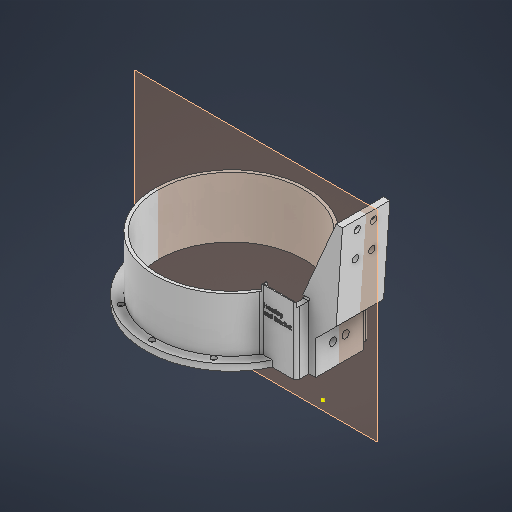
# Autodesk Inventor part: Holder_and_Cylinder
Saved by Autodesk Inventor 2026 (Build 300175000, 175)
## iProperties
Created: 2025-06-26
Part Number: Holder_and_Cylinder
Material: Generic
Document SubType Name: Modeling
Designer: Charl
Density: 1 g/cm^3
Appearance: Default
Author: Charl
Autodesk Inventor part; units mm, degrees
(part 1 of 2)
ref_plane "YZ Plane" through (0, 0, 0) normal (1, 0, 0) x (0, 1, 0)
ref_plane "XZ Plane" through (0, 0, 0) normal (0, 1, 0) x (-1, 0, 0)
ref_plane "XY Plane" through (0, 0, 0) normal (0, 0, 1) x (1, 0, 0)
sketch "Sketch1" plane through (0, 0, 0) normal (0, 1, 0) x (-1, 0, 0)
  circle A0 centre (0, 0) radius 135
  circle A1 centre (0, 0) radius 120
  dimension "d0" = 270
  dimension "d1" = 240
  constraints: 2 centre point, 2 coincident
  measures "d0" diameter of A0
  measures "d1" diameter of A1
extrude "Extrusion1" add sketch "Sketch1" along normal blind 10
sketch "Sketch2" plane through (0, 10, 0) normal (0, 1, 0) x (1, 0, 0)
  circle A0 centre (0, 0) radius 115.125
  circle A1 centre (0, 0) radius 120
  dimension "d4" = 230.25
  constraints: 2 centre point, 2 coincident
  measures "d4" diameter of A0
extrude "Extrusion2" add sketch "Sketch2" along normal blind 85.5 and the other way blind 10
sketch "Sketch3" plane through (0, 10, 0) normal (0, 1, 0) x (1, 0, 0)
  line L0 (70.125, 57.5) -> (160.125, 57.5)
  line L1 (160.125, 57.5) -> (160.125, -57.5)
  line L2 (160.125, -57.5) -> (70.125, -57.5)
  line L3 (70.125, -57.5) -> (70.125, 57.5)
  line L4 (71.625, 56) -> (158.625, 56)
  line L5 (158.625, 56) -> (158.625, -56)
  line L6 (158.625, -56) -> (71.625, -56)
  line L7 (71.625, -56) -> (71.625, 56)
  line L8 (-160.125, 32.5) -> (-70.125, 32.5)
  line L9 (-70.125, 32.5) -> (-70.125, -32.5)
  line L10 (-70.125, -32.5) -> (-160.125, -32.5)
  line L11 (-160.125, -32.5) -> (-160.125, 32.5)
  line L12 (-158.625, 31) -> (-71.625, 31)
  line L13 (-71.625, 31) -> (-71.625, -31)
  line L14 (-71.625, -31) -> (-158.625, -31)
  line L15 (-158.625, -31) -> (-158.625, 31)
  line L16 (-150.359, 85.157) -> (-65.125, 85.157)
  line L17 (-65.125, 85.157) -> (-65.125, 46.3)
  line L18 (-65.125, 46.3) -> (-150.359, 46.3)
  line L19 (-150.359, 46.3) -> (-150.359, 85.157)
  line L20 (-148.359, 83.157) -> (-67.125, 83.157)
  line L21 (-67.125, 83.157) -> (-67.125, 48.3)
  line L22 (-67.125, 48.3) -> (-148.359, 48.3)
  line L23 (-148.359, 48.3) -> (-148.359, 83.157)
  line L24 (-150.359, -46.3) -> (-65.125, -46.3)
  line L25 (-65.125, -46.3) -> (-65.125, -85.157)
  line L26 (-65.125, -85.157) -> (-150.359, -85.157)
  line L27 (-150.359, -85.157) -> (-150.359, -46.3)
  line L28 (-148.359, -48.3) -> (-67.125, -48.3)
  line L29 (-67.125, -48.3) -> (-67.125, -83.157)
  line L30 (-67.125, -83.157) -> (-148.359, -83.157)
  line L31 (-148.359, -83.157) -> (-148.359, -48.3)
  circle A0 centre (0, 0) radius 134.272
  circle A1 centre (0, 0) radius 132.2722
  circle A2 centre (0, 0) radius 115.125
  circle A3 centre (0, 0) radius 120
  point P0 (70.125, 0)
  point P1 (121.3372, 57.5)
  point P2 (122.0368, 56)
  point P3 (122.0368, -56)
  point P4 (121.3372, -57.5)
  point P5 (106.132, 56)
  point P6 (100.5871, 56)
  point P7 (100.5871, -56)
  point P8 (106.132, -56)
  point P9 (105.3269, 57.5)
  point P10 (105.3269, -57.5)
  dimension "d7" = 90
  dimension "d8" = 115
  dimension "d9" = 57.5
  dimension "d10" = 70.125
  dimension "d11" = 1.5
  dimension "d12" = 1.5
  dimension "d13" = 1.5
  dimension "d14" = 1.5
  dimension "d15" = 90
  dimension "d16" = 65
  dimension "d17" = 32.5
  dimension "d18" = 70.125
  dimension "d19" = 1.5
  dimension "d20" = 1.5
  dimension "d21" = 1.5
  dimension "d22" = 1.5
  dimension "d23" = 85.234
  dimension "d24" = 38.857
  dimension "d25" = 2
  dimension "d26" = 2
  dimension "d27" = 2
  dimension "d28" = 2
  dimension "d29" = 65.125
  dimension "d30" = 13.8
  dimension "d31" = 13.8
  dimension "d32" = 65.125
  dimension "d33" = 38.857
  dimension "d34" = 85.234
  dimension "d35" = 2
  dimension "d36" = 2
  dimension "d37" = 2
  dimension "d38" = 2
  dimension "d39" = 268.544
  dimension "d40" = 264.5444
  dimension "d42" = 230.25
  dimension "d45" = 240
  constraints: 64 end point, 16 parallel, 8 horizontal, 8 perpendicular, 4 centre point, 3 coincident, 1 midpoint
  measures "d7" distance of L0.start L0.end
  measures "d8" distance of L0.end L1.end
  measures "d9" distance from line of point (0, 0) L0
  measures "d10" distance of point (70.125, 0) point (0, 0)
  measures "d11" distance between parallel lines of L1 L5
  measures "d12" distance between parallel lines of L2 L6
  measures "d13" distance between parallel lines of L0 L4
  measures "d14" distance between parallel lines of L3 L7
  measures "d15" distance of L8.start L8.end
  measures "d16" distance of L8.end L9.end
  measures "d17" distance from line of point (0, 0) L8
  measures "d18" distance from line of L9 point (0, 0)
  measures "d19" distance between parallel lines of L10 L14
  measures "d20" distance between parallel lines of L9 L13
  measures "d21" distance between parallel lines of L8 L12
  measures "d22" distance between parallel lines of L11 L15
  measures "d23" distance of L17.end L18.end
  measures "d24" distance of L16.end L17.end
  measures "d25" distance between parallel lines of L16 L20
  measures "d26" distance between parallel lines of L19 L23
  measures "d27" distance between parallel lines of L18 L22
  measures "d28" distance between parallel lines of L17 L21
  measures "d29" distance from line of point (0, 0) L17
  measures "d30" distance from line of L8 L18.end
  measures "d31" distance between parallel lines of L10 L24
  measures "d32" distance from line of point (0, 0) L25
  measures "d33" distance of L26.end L24.start
  measures "d34" distance of L25.end L26.end
  measures "d35" distance between parallel lines of L27 L31
  measures "d36" distance between parallel lines of L24 L28
  measures "d37" distance between parallel lines of L25 L29
  measures "d38" distance between parallel lines of L26 L30
  measures "d39" diameter of A0
  measures "d40" diameter of A1
  measures "d42" diameter of A2
  measures "d45" diameter of A3
extrude "Extrusion3" cut sketch "Sketch3" along normal mid plane 85.5 contours L0 L1 L2 A0 L6 L5 L4
extrude "Extrusion4" cut sketch "Sketch3" along normal blind 85.5 contours L4 A3 L6 A2
extrude "Extrusion5" add sketch "Sketch3" along normal blind 85.5 and the other way blind 10 contours L0 A1 L4 A3 | L0 A0 L4 A1 | A3 L6 A1 L2 | L0 L1 L2 A0 L6 L5 L4 | A1 L6 A0 L2
sketch "Sketch5" plane through (0, 0, 0) normal (0, -1, 0) x (1, 0, 0)
  line L0 (135, -56) -> (160, -56)
  line L1 (160, -56) -> (160, 56)
  line L2 (160, 56) -> (135, 56)
  line L3 (135, 56) -> (135, -56)
  arc A0 (122.8373, -56) -> (122.8373, 56) centre (0, 0) ccw projected
  dimension "d57" = 25
  dimension "d58" = 112
  dimension "d59" = 56
  constraints: 8 end point, 2 parallel, 1 horizontal, 1 perpendicular, 1 tangent
  measures "d57" distance of L0.start L0.end
  measures "d58" distance of L2.end L0.start
  measures "d59" distance from line of point (0, 0) L0
extrude "Extrusion7" add sketch "Sketch5" against normal blind 80
chamfer "Chamfer1" distance 40 angle 23.25 1 edges at (135, 80, 0) measured on face at (135, 79.5, 0)
ref_plane "Work Plane1" through (105.3269, 10, 0) normal (0, 0, 1) x (1, 0, 0)
sketch "Sketch6" plane through (135, 40, -56) normal (-0.9187912, 0.3947439, 0) x (0, 0, 1)
  circle A0 centre (56, 33.7805) radius 5.5
  circle A1 centre (56, 33.7805) radius 2
  circle A2 centre (46, 10.0805) radius 5.5
  circle A3 centre (46, 10.0805) radius 2
  line L0 (56, 109.6115) -> (56, -231.2929) projected
  line L1 (112, 43.5355) -> (0, 43.5355) projected
  circle A4 centre (66, 10.0805) radius 5.5
  circle A5 centre (66, 10.0805) radius 2
  point P0 (56, -90.0421)
  dimension "d65" = 11
  dimension "d66" = 4
  dimension "d67" = 11
  dimension "d68" = 4
  dimension "d69" = 10
  dimension "d70" = 23.7
  dimension "d71" = 9.755
  dimension "d72" = 11
  dimension "d73" = 4
  dimension "d76" = 23.7
  dimension "d77" = 10
  constraints: 6 centre point, 3 coincident
  measures "d65" diameter of A0
  measures "d66" diameter of A1
  measures "d67" diameter of A2
  measures "d68" diameter of A3
  measures "d69" distance from line of L0 A2.centre
  measures "d70" vertical distance of A0.centre A2.centre
  measures "d71" distance from line of L1 A0.centre
  measures "d72" diameter of A4
  measures "d73" diameter of A5
  measures "d76" vertical distance of A0.centre A4.centre
  measures "d77" distance from line of A5.centre L0
extrude "Extrusion8" cut sketch "Sketch6" against normal blind 55 contours A0 L0 A1 | L0 A1 A0 | L0 A1 | A1 L0 | A2 | A3 | A4 | A5
extrude "Extrusion9" add sketch "Sketch6" against normal blind 5 contours A0 L0 A1 | L0 A1 A0 | A2 | A4
sketch "Sketch17" plane through (160.125, 0, -57.5) normal (1, 0, 0) x (0, 0, -1)
  line L0 (-95, 111) -> (-20, 111)
  line L1 (-20, 111) -> (-20, 76)
  line L2 (-20, 76) -> (-95, 76)
  line L3 (-95, 76) -> (-95, 111)
  line L4 (-115, 0) -> (-115, 95.5) projected
  line L5 (-115, 95.5) -> (0, 95.5) projected
  point P0 (-57.5, 0)
  dimension "d130" = 20
  dimension "d131" = 35
  dimension "d132" = 19.5
  dimension "d133" = 75
  constraints: 8 end point, 2 parallel, 1 horizontal, 1 perpendicular
  measures "d130" distance between parallel lines of L4 L3
  measures "d131" distance between parallel lines of L2 L0
  measures "d132" distance between parallel lines of L5 L2
  measures "d133" distance between parallel lines of L1 L3
extrude "Extrusion16" cut sketch "Sketch17" against normal blind 40.5
sketch "Sketch18" plane through (0, 95.5, 0) normal (0, 1, 0) x (1, 0, 0)
  line L0 (100.5871, 56) -> (158.625, 56) projected
  line L1 (152.1854, 37.5) -> (152.1854, 56) projected
  line L2 (158.625, 56) -> (152.1854, 56)
  line L3 (152.1854, 56) -> (152.1854, 37.5)
  line L4 (152.1854, 37.5) -> (158.625, 37.5)
  line L5 (158.625, 37.5) -> (158.625, 56)
  line L6 (160.125, -37.5) -> (150.4668, -37.5) projected
  line L7 (158.625, -56) -> (100.5871, -56) projected
  line L8 (152.1854, -37.5) -> (158.625, -37.5)
  line L9 (158.625, -37.5) -> (158.625, -56)
  line L10 (158.625, -56) -> (152.1854, -56)
  line L11 (152.1854, -56) -> (152.1854, -37.5)
  point P0 (0, 0)
  constraints: 16 end point, 4 parallel, 2 horizontal, 2 perpendicular, 2 point on line
extrude "Extrusion17" add sketch "Sketch18" against normal blind 40.5
sketch "Sketch19" plane through (0, 95.5, 0) normal (0, 1, 0) x (1, 0, 0)
  arc A0 (105.3269, 57.5) -> (105.3269, -57.5) centre (0, 0) ccw projected
  line L0 (152.1854, 56) -> (135, 56) projected
  line L1 (106.132, 56) -> (152.1854, 56)
  line L2 (106.132, 56) -> (106.132, 57.5)
  line L3 (105.3269, 57.5) -> (122.1423, 57.5) projected
  line L4 (160.125, 57.5) -> (160.125, -57.5) projected
  line L5 (106.132, 57.5) -> (160.125, 57.5)
  line L6 (160.125, 57.5) -> (160.125, -57.5)
  line L7 (160.125, -57.5) -> (106.132, -57.5)
  line L8 (106.132, -57.5) -> (106.132, -56)
  line L9 (135, -56) -> (152.1854, -56) projected
  line L10 (152.1854, -56) -> (106.132, -56)
  line L11 (152.1854, -37.5) -> (150.4668, -37.5) projected
  line L12 (152.1854, -56) -> (152.1854, -37.5)
  line L13 (152.1854, -37.5) -> (160.125, -37.5)
  line L14 (122.726, 57.5) -> (142.726, 57.5)
  line L15 (142.726, 57.5) -> (142.726, 56)
  line L16 (142.726, 56) -> (122.726, 56)
  line L17 (122.726, 56) -> (122.726, 57.5)
  line L18 (152.1854, 56) -> (152.1854, 37.5) projected
  line L19 (152.1854, 56) -> (152.1854, 37.5)
  line L20 (152.1854, 37.5) -> (160.125, 37.5)
  dimension "d138" = 20
  dimension "d139" = 17.399
  constraints: 30 end point, 6 point on line, 5 perpendicular, 3 horizontal, 3 vertical, 2 collinear, 2 parallel
  measures "d138" distance of L15.end L16.end
  measures "d139" distance between parallel lines of L4 L15
extrude "Extrusion18" add sketch "Sketch19" along normal blind 4 contours L0 L15 L5 L4 L20 L18 | L1 L2 L3 L5 L17 | L4 L7 L8 L10 L9 L12 L13
sketch "Sketch20" plane through (122.8373, 10, 56) normal (0, 0, -1) x (-1, 0, 0)
  line L0 (-29.3481, 89.5) -> (-29.3481, 70) projected
  line L1 (16.7053, 85.5) -> (16.7053, 89.5) projected
  line L2 (-29.3481, 89.5) -> (16.7053, 89.5)
  line L3 (16.7053, 89.5) -> (16.7053, 88)
  line L4 (16.7053, 88) -> (-29.3481, 88)
  line L5 (-29.3481, 88) -> (-29.3481, 89.5)
  point P0 (122.8373, -10)
  dimension "d142" = 1.5
  constraints: 8 end point, 2 parallel, 1 horizontal, 1 perpendicular, 1 point on line
  measures "d142" distance of L2.end L3.end
extrude "Extrusion19" add sketch "Sketch20" along normal blind 5
sketch "Sketch21" plane through (0, 99.5, 0) normal (0, 1, 0) x (1, 0, 0)
  line L0 (106.132, 57.5) -> (106.132, 56) projected
  line L1 (106.132, 57.5) -> (107.632, 57.5)
  line L2 (107.632, 57.5) -> (107.632, 51)
  line L3 (107.632, 51) -> (106.132, 51)
  line L4 (106.132, 51) -> (106.132, 57.5)
  line L5 (160.125, -57.5) -> (122.1423, -57.5) projected
  line L6 (106.132, -56) -> (106.132, -51) projected
  line L7 (160.125, -57.5) -> (106.132, -57.5)
  line L8 (106.132, -57.5) -> (106.132, -56)
  line L9 (106.132, -56) -> (160.125, -56)
  line L10 (160.125, -56) -> (160.125, -57.5)
  point P0 (0, 0)
  dimension "d145" = 1.5
  dimension "d146" = 6.5
  dimension "d147" = 1.5
  constraints: 16 end point, 4 parallel, 2 horizontal, 2 perpendicular
  measures "d145" distance of L2.end L3.end
  measures "d146" distance of L1.end L2.end
  measures "d147" distance of L7.end L6.start
extrude "Extrusion20" add sketch "Sketch21" along normal blind 6.5
sketch "Sketch22" plane through (160.125, 99.5, 56) normal (0, 0, -1) x (-1, 0, 0)
  line L0 (412.3732, -43.6088) -> (412.3732, -42.1088)
  line L1 (412.3732, -42.1088) -> (412.3732, -42.1088)
  line L2 (0, -99.5) -> (0, 6.5) projected
  line L3 (53.993, -4) -> (53.993, 6.5) projected
  line L4 (0, 6.5) -> (53.993, 6.5)
  line L5 (53.993, 6.5) -> (53.993, 5)
  line L6 (53.993, 5) -> (0, 5)
  line L7 (0, 5) -> (0, 6.5)
  line L8 (53.993, 0) -> (0, 0) projected
  line L9 (53.993, 6.5) -> (52.493, 6.5)
  line L10 (52.493, 6.5) -> (52.493, 0)
  line L11 (52.493, 0) -> (53.993, 0)
  line L12 (53.993, 0) -> (53.993, 6.5)
  point P0 (160.125, -99.5)
  dimension "d150" = 1.5
  dimension "d151" = 1.5
  dimension "d152" = 1.5
  constraints: 20 end point, 4 parallel, 3 horizontal, 2 perpendicular, 2 point on line, 2 vertical, 5 other
  measures "d150" distance of L0.end L0.start
  measures "d151" distance of L4.end L5.end
  measures "d152" distance of L11.end L10.end
extrude "Extrusion21" add sketch "Sketch22" along normal blind 5 contours L10 L6 L3 L8 | L10 L4 L3 L6
sketch "Sketch23" plane through (106.132, 10, -56) normal (0, 0, 1) x (1, 0, 0)
  line L0 (16.594, 85.5) -> (16.594, 89.5) projected
  line L1 (0, 85.5) -> (0, 89.5) projected
  line L2 (16.594, 89.5) -> (0, 89.5)
  line L3 (0, 89.5) -> (0, 88)
  line L4 (0, 88) -> (16.594, 88)
  line L5 (16.594, 88) -> (16.594, 89.5)
  line L6 (36.594, 89.5) -> (46.0534, 89.5) projected
  line L7 (46.0534, 70) -> (46.0534, 89.5) projected
  line L8 (36.594, 89.5) -> (46.0534, 89.5)
  line L9 (46.0534, 89.5) -> (46.0534, 88)
  line L10 (46.0534, 88) -> (36.594, 88)
  line L11 (36.594, 88) -> (36.594, 89.5)
  point P0 (-106.132, -10)
  dimension "d155" = 1.5
  dimension "d156" = 1.5
  constraints: 16 end point, 4 parallel, 2 horizontal, 2 perpendicular, 2 point on line
  measures "d155" distance of L3.end L2.end
  measures "d156" distance of L8.end L9.end
extrude "Extrusion22" add sketch "Sketch23" along normal blind 5
sketch "Sketch24" plane through (107.632, 99.5, -51) normal (1, 0, 0) x (0, 0, -1)
  line L0 (0, 0) -> (0, 6.5) projected
  line L1 (6.5, 0) -> (6.5, 6.5) projected
  line L2 (0, 6.5) -> (6.5, 6.5)
  line L3 (6.5, 6.5) -> (6.5, 5)
  line L4 (6.5, 5) -> (0, 5)
  line L5 (0, 5) -> (0, 6.5)
  point P0 (-51, -99.5)
  point P1 (0, 5)
  dimension "d159" = 1.5
  constraints: 8 end point, 2 parallel, 1 horizontal, 1 perpendicular, 1 point on line
  measures "d159" distance of L2.end L3.end
extrude "Extrusion23" add sketch "Sketch24" along normal blind 5
fillet "Fillet2" radius 5 6 edges at (100.5871, 52.75, 56) (100.5871, 52.75, -56) (105.3269, 52.75, -57.5) (105.3269, 52.75, 57.5) (160.125, 49.75, -57.5) (160.125, 53, 57.5)
chamfer "Chamfer2" distance 4 angle 45 2 edges at (129.1587, 98, 56) (152.1854, 98, 53.5)
ref_plane "Work Plane2" through (135, 0, 56) normal (-0.4107189, -0.911762, 0) x (0, 0, -1)
sketch "Sketch27" plane through (0, 0, 0) normal (0, -1, 0) x (1, 0, 0)
  line L0 (152.1854, 51) -> (152.1854, 56) projected
  line L1 (122.726, -56) -> (106.132, -56) projected
  line L2 (152.1854, 56) -> (121.3527, 56)
  line L3 (121.3527, 56) -> (121.3527, -56)
  line L4 (121.3527, -56) -> (152.1854, -56)
  line L5 (152.1854, -56) -> (152.1854, 56)
  point P0 (0, 0)
  constraints: 8 end point, 2 parallel, 1 horizontal, 1 perpendicular, 1 point on line
extrude "Extrusion25" add sketch "Sketch27" against normal blind 10
sketch "Sketch25" plane through (135, 0, 56) normal (-0.4107189, -0.911762, 0) x (0, 0, -1)
  line L0 (18.5, -17.1126) -> (93.5, -17.1126) projected
  circle A0 centre (56, -31.1821) radius 20
  ellipse E0 centre (56, -127.1951) end of major axis (-59.125, -127.1951) minor radius 104.9666 (114.461, -36.7692) -> (-2.461, -36.7692) ccw projected
  point P0 (56, -123.0879)
  dimension "d170" = 40
  dimension "d172" = 96.013
  constraints: 1 centre point, 1 other
  measures "d170" diameter of A0
  measures "d172" distance of point (56, -127.195) A0.centre
extrude "Extrusion24" cut sketch "Sketch25" along normal mid plane 80
sketch "Sketch28" plane through (0, 10, 0) normal (0, 1, 0) x (1, 0, 0)
  circle A0 centre (0, 0) radius 125
  circle A1 centre (0, 0) radius 135
  circle A2 centre (0, 125) radius 2.75
  circle A3 centre (0, 125) radius 4.35
  dimension "d177" = 250
  dimension "d178" = 270
  dimension "d179" = 5.5
  dimension "d180" = 8.7
  constraints: 3 centre point, 3 coincident, 1 vertical alignment, 2 other
  measures "d178" diameter of A1
  measures "d179" diameter of A2
  measures "d180" diameter of A3
extrude "Extrusion26" cut sketch "Sketch28" against normal blind 5 contours A3 A0 A2 | A0 A2 A3 | A2 A0 | A0 A2
extrude "Extrusion27" cut sketch "Sketch28" against normal blind 10 contours A2 A0 | A0 A2
pattern_circular "Circular Pattern1" count 10 over 360 about axis through (0, 0, 0) along (0, 1, 0) of "Extrusion26", "Extrusion27"
sketch "Sketch29" plane through (160.125, 76, 37.5) normal (0, 1, 0) x (1, 0, 0)
  line L0 (-9.6582, 75) -> (-7.9396, 75) projected
  line L1 (-9.6582, 75) -> (10.6418, 75)
  line L2 (10.6418, 75) -> (10.6418, 0)
  line L3 (10.6418, 0) -> (-9.6582, 0)
  line L4 (-9.6582, 0) -> (-9.6582, 75)
  point P0 (-160.125, 37.5)
  point P1 (-7.9396, 75)
  dimension "d188" = 75
  dimension "d189" = 20.3
  constraints: 8 end point, 2 parallel, 1 horizontal, 1 perpendicular
  measures "d188" distance of L1.end L2.end
  measures "d189" distance of L2.end L3.end
extrude "HolderStart" add sketch "Sketch29" along normal blind 10 separate body
sketch "Sketch31" plane through (160.125, 76, 37.5) normal (0, -1, 0) x (1, 0, 0)
  line L0 (-9.6582, 0) -> (10.6418, 0) projected
  line L1 (0, -75) -> (0, 0) projected
  line L2 (10.6418, 0) -> (0, 0)
  line L3 (0, 0) -> (0, -75)
  line L4 (0, -75) -> (10.6418, -75)
  line L5 (10.6418, -75) -> (10.6418, 0)
  point P0 (-160.125, -37.5)
  constraints: 8 end point, 2 parallel, 1 horizontal, 1 perpendicular
extrude "Extrusion30" add sketch "Sketch31" along normal blind 76 bodies 2
sketch "Sketch32" plane through (150.4668, 86, 37.5) normal (0, 0, 1) x (1, 0, 0)
  line L0 (20.3, -86) -> (20.3, 0) projected
  line L1 (52.705, 0) -> (115.8158, 0) construction
  line L2 (0, 0) -> (20.3, 0) projected
  line L3 (0, 0) -> (0, 13.494)
  line L4 (8.2289, 20) -> (-42.8348, 20) projected
  line L5 (0, 13.494) -> (10, 13.494)
  line L6 (10, 13.494) -> (10, 17.494)
  line L7 (10, 17.494) -> (0, 17.494)
  line L8 (20.3, -32.405) -> (52.705, 0)
  line L9 (0, 17.494) -> (14.8386, 52.0317)
  line L10 (14.8386, 52.0317) -> (16.9363, 56.9144)
  line L11 (52.705, 0) -> (52.705, 74.2114) construction
  line L12 (52.705, 74.2114) -> (52.705, 193.2478) construction
  line L13 (16.9363, 56.9144) -> (52.705, 140.1682)
  line L14 (52.705, 116.8926) -> (42.705, 116.8926)
  line L15 (42.705, 116.8926) -> (42.705, 116.8926) construction
  line L16 (52.705, 116.8926) -> (62.705, 116.8926) construction
  line L17 (62.705, 116.8926) -> (134.3375, 116.8926) construction
  line L18 (52.705, 140.1682) -> (62.705, 140.1682)
  line L19 (62.705, 140.1682) -> (52.705, 0)
  point P0 (-150.4668, -86)
  dimension "d200" = 13.494
  dimension "d201" = 4
  dimension "d211" = 45
  dimension "d212" = 0
  dimension "d213" = 32.405
  dimension "d239" = 10
  dimension "d240" = 10
  dimension "d241" = 66.75
  dimension "d244" = 10
  dimension "d245" = 0
  dimension "d246" = 66.75
  dimension "d247" = 10
  constraints: 34 end point, 6 perpendicular, 5 point on line, 3 horizontal, 2 vertical
  measures "d200" distance of L2.start L3.end
  measures "d201" distance of L5.end L6.end
  measures "d211" angle of L8 L0
  measures "d212" vertical distance of L0.end L1.start
  measures "d213" distance of L0.end L8.start
  measures "d239" distance of L6.end L7.end
  measures "d240" distance of L3.end L5.end
  measures "d241" angle of L7 L9
  measures "d244" distance of L14.start L14.end
  measures "d245" distance of L14.end L15.end
  measures "d246" angle of L1 L13
  measures "d247" distance of L14.start L16.end
extrude "Extrusion35" add sketch "Sketch32" against normal blind 75 bodies 2
ref_plane "Work Plane7" through (150.4668, 103.494, 37.5) normal (0.3947439, 0.9187912, 0) x (0, 0, -1)
sketch "Sketch35" plane through (150.4668, 103.494, 37.5) normal (0.3947439, 0.9187912, 0) x (0, 0, -1)
  line L0 (0, 0) -> (75, 0) projected
  circle A0 centre (37.5, 15) radius 35
  point P0 (37.5, 97.394)
  dimension "d252" = 70
  dimension "d253" = 15
  constraints: 1 centre point
  measures "d252" diameter of A0
  measures "d253" distance from line of L0 A0.centre
extrude "Extrusion36" cut sketch "Sketch35" along normal blind 67.371 and the other way blind 65.75 bodies 2
ref_plane "Work Plane9" through (166.2261, 2.0933, -37.5) normal (-0.9081432, 0.4186597, 0) x (0, 0, 1)
ref_plane "Work Plane8" through (170.7668, 0, -37.5) normal (-0.9081432, 0.4186597, 0) x (0, 0, 1)
sketch "Sketch36" plane through (166.2261, 2.0933, -37.5) normal (-0.9081432, 0.4186597, 0) x (0, 0, 1)
  circle A0 centre (50.5, 208.9598) radius 2
  circle A1 centre (50.5, 208.9598) radius 5
  circle A2 centre (50.5, 169.9598) radius 2
  circle A3 centre (50.5, 169.9598) radius 5
  line L0 (75, 91.667) -> (0, 91.667) construction
  line L1 (37.5, -67.9361) -> (37.5, 251.2701) construction
  circle A4 centre (24.5, 208.9598) radius 2
  circle A5 centre (24.5, 208.9598) radius 5
  circle A6 centre (24.5, 169.9598) radius 2
  circle A7 centre (24.5, 169.9598) radius 5
  line L2 (75, 223.1464) -> (0, 223.1464) projected
  line L3 (75, 218.9598) -> (0, 218.9598) projected
  point P0 (37.5, -71.4932)
  point P1 (37.5, 91.667)
  dimension "d260" = 10
  dimension "d261" = 4
  dimension "d262" = 10
  dimension "d263" = 4
  dimension "d264" = 39
  dimension "d266" = 26
  dimension "d267" = 10
  dimension "d268" = 26
  constraints: 8 centre point, 4 coincident, 4 symmetric about line, 2 end point, 2 midpoint, 1 vertical, 4 other
  measures "d260" diameter of A1
  measures "d261" diameter of A0
  measures "d262" diameter of A3
  measures "d263" diameter of A2
  measures "d264" distance of A2.centre A0.centre
  measures "d266" distance of A5.centre A0.centre
  measures "d267" distance from line of L3 A0.centre
  measures "d268" distance of A7.centre A2.centre
extrude "Extrusion37" cut sketch "Sketch36" along normal blind 49 contours A0 | A1 | A2 | A3 | A4 | A5 | A6 | A7 bodies 2
extrude "Extrusion38" cut sketch "Sketch36" along normal blind 75 contours A0 | A2 | A4 | A6 bodies 2
ref_plane "Work Plane10" through (196.4064, 56.2628, -37.5) normal (-0.9187912, 0.3947439, 0) x (0, 0, 1)
sketch "Sketch37" plane through (196.4064, 56.2628, -37.5) normal (-0.9187912, 0.3947439, 0) x (0, 0, 1)
  point P0 (37.5, -129.224)
sketch "Sketch38" plane through (196.4064, 56.2628, -37.5) normal (-0.9187912, 0.3947439, 0) x (0, 0, 1)
  circle A0 centre (47.5, -29.1015) radius 5.5 projected
  circle A1 centre (27.5, -29.1015) radius 5.5 projected
  circle A2 centre (37.5, -5.4015) radius 5.5 projected
  circle A3 centre (27.5, -29.1015) radius 5.5
  circle A4 centre (47.5, -29.1015) radius 5.5
  circle A5 centre (37.5, -5.4015) radius 5.5
  point P0 (37.5, -129.224)
  constraints: 3 centre point, 3 coincident, 3 concentric
extrude "Extrusion39" cut sketch "Sketch38" along normal blind 44.5 bodies 2
sketch "Sketch39" plane through (122.1423, 0, 57.5) normal (0, 0, 1) x (1, 0, 0)
  line L0 (-13.5441, 81.6413) -> (29.5653, 81.6413) construction
  line L1 (29.5653, 81.6413) -> (29.5653, 47.1733) construction
  line L2 (29.5653, 47.1733) -> (-13.5441, 47.1733) construction
  line L3 (-13.5441, 47.1733) -> (-13.5441, 81.6413) construction
  line L4 (-8.497, 75.5017) -> (-9.3077, 75.5017)
  line L5 (-9.3077, 75.5017) -> (-9.3077, 78.4875)
  line L6 (-9.3077, 78.4875) -> (-12.1155, 78.4875)
  line L7 (-12.1155, 78.4875) -> (-12.1155, 75.5017)
  line L8 (-12.1155, 75.5017) -> (-12.9262, 75.5017)
  line L9 (-12.9262, 75.5017) -> (-12.9262, 81.6017)
  line L10 (-12.9262, 81.6017) -> (-12.1155, 81.6017)
  line L11 (-12.1155, 81.6017) -> (-12.1155, 79.2092)
  line L12 (-12.1155, 79.2092) -> (-9.3077, 79.2092)
  line L13 (-9.3077, 79.2092) -> (-9.3077, 81.6017)
  line L14 (-9.3077, 81.6017) -> (-8.497, 81.6017)
  line L15 (-8.497, 81.6017) -> (-8.497, 75.5017)
  spline S0 degree 2 poles (-3.5587, 77.7905) (-3.5587, 76.6337) (-4.6709, 75.3732) (-5.6002, 75.3732) knots 0 0 0 1 2 2 2
  spline S1 degree 2 poles (-5.6002, 75.3732) (-6.5543, 75.3732) (-7.6468, 76.6733) (-7.6468, 77.7905) knots 0 0 0 1 2 2 2
  spline S2 degree 2 poles (-7.6468, 77.7905) (-7.6468, 78.9373) (-6.5197, 80.2077) (-5.6002, 80.2077) knots 0 0 0 1 2 2 2
  spline S3 degree 2 poles (-5.6002, 80.2077) (-4.6709, 80.2077) (-3.5587, 78.9423) (-3.5587, 77.7905) knots 0 0 0 1 2 2 2
  spline S4 degree 2 poles (-4.3545, 77.7905) (-4.3545, 78.6803) (-5.0021, 79.5453) (-5.6002, 79.5453) knots 0 0 0 1 2 2 2
  spline S5 degree 2 poles (-5.6002, 79.5453) (-6.1984, 79.5453) (-6.8509, 78.6803) (-6.8509, 77.7905) knots 0 0 0 1 2 2 2
  spline S6 degree 2 poles (-6.8509, 77.7905) (-6.8509, 76.9254) (-6.1984, 76.0356) (-5.6002, 76.0356) knots 0 0 0 1 2 2 2
  spline S7 degree 2 poles (-5.6002, 76.0356) (-5.007, 76.0356) (-4.3545, 76.9106) (-4.3545, 77.7905) knots 0 0 0 1 2 2 2
  line L16 (0.7914, 75.5017) -> (0.0203, 75.5017)
  line L17 (0.0203, 75.5017) -> (0.0203, 76.0059)
  spline S8 degree 2 poles (0.0203, 76.0059) (-0.3357, 75.6945) (-0.9733, 75.3732) (-1.3688, 75.3732) knots 0 0 0 1 2 2 2
  spline S9 degree 2 poles (-1.3688, 75.3732) (-1.6654, 75.3732) (-2.1943, 75.5709) (-2.3871, 75.7835) knots 0 0 0 1 2 2 2
  spline S10 degree 2 poles (-2.3871, 75.7835) (-2.5848, 75.9961) (-2.8023, 76.6436) (-2.8023, 77.1083) knots 0 0 0 1 2 2 2
  line L18 (-2.8023, 77.1083) -> (-2.8023, 80.0792)
  line L19 (-2.8023, 80.0792) -> (-2.0312, 80.0792)
  line L20 (-2.0312, 80.0792) -> (-2.0312, 77.4692)
  spline S11 degree 2 poles (-2.0312, 77.4692) (-2.0312, 77.1034) (-1.9768, 76.6239) (-1.8829, 76.4459) knots 0 0 0 1 2 2 2
  spline S12 degree 2 poles (-1.8829, 76.4459) (-1.789, 76.2679) (-1.4677, 76.1048) (-1.1661, 76.1048) knots 0 0 0 1 2 2 2
  spline S13 degree 2 poles (-1.1661, 76.1048) (-0.8844, 76.1048) (-0.2467, 76.4261) (0.0203, 76.6585) knots 0 0 0 1 2 2 2
  line L21 (0.0203, 76.6585) -> (0.0203, 80.0792)
  line L22 (0.0203, 80.0792) -> (0.7914, 80.0792)
  line L23 (0.7914, 80.0792) -> (0.7914, 75.5017)
  spline S14 degree 2 poles (3.1444, 75.393) (2.6847, 75.393) (1.8888, 75.6401) (1.6268, 75.7786) knots 0 0 0 1 2 2 2
  line L24 (1.6268, 75.7786) -> (1.6268, 76.6436)
  line L25 (1.6268, 76.6436) -> (1.6664, 76.6436)
  spline S15 degree 2 poles (1.6664, 76.6436) (1.7652, 76.5645) (2.0322, 76.3767) (2.2546, 76.2729) knots 0 0 0 1 2 2 2
  spline S16 degree 2 poles (2.2546, 76.2729) (2.4474, 76.179) (2.922, 76.0405) (3.1741, 76.0405) knots 0 0 0 1 2 2 2
  spline S17 degree 2 poles (3.1741, 76.0405) (3.357, 76.0405) (3.7771, 76.1246) (3.876, 76.1938) knots 0 0 0 1 2 2 2
  spline S18 degree 2 poles (3.876, 76.1938) (4.0194, 76.2877) (4.1479, 76.5003) (4.1479, 76.7178) knots 0 0 0 1 2 2 2
  spline S19 degree 2 poles (4.1479, 76.7178) (4.1479, 76.9897) (3.8513, 77.2714) (3.4707, 77.3653) knots 0 0 0 1 2 2 2
  spline S20 degree 2 poles (3.4707, 77.3653) (3.3224, 77.3999) (2.8478, 77.4988) (2.6451, 77.5532) knots 0 0 0 1 2 2 2
  spline S21 degree 2 poles (2.6451, 77.5532) (2.1212, 77.7064) (1.6466, 78.3392) (1.6466, 78.789) knots 0 0 0 1 2 2 2
  spline S22 degree 2 poles (1.6466, 78.789) (1.6466, 79.4119) (2.5809, 80.188) (3.352, 80.188) knots 0 0 0 1 2 2 2
  spline S23 degree 2 poles (3.352, 80.188) (3.7327, 80.188) (4.5038, 80.0001) (4.7658, 79.8568) knots 0 0 0 1 2 2 2
  line L26 (4.7658, 79.8568) -> (4.7658, 79.0312)
  line L27 (4.7658, 79.0312) -> (4.7263, 79.0312)
  spline S24 degree 2 poles (4.7263, 79.0312) (4.4297, 79.2685) (3.7079, 79.5404) (3.3372, 79.5404) knots 0 0 0 1 2 2 2
  spline S25 degree 2 poles (3.3372, 79.5404) (2.9566, 79.5404) (2.4326, 79.2191) (2.4326, 78.8978) knots 0 0 0 1 2 2 2
  spline S26 degree 2 poles (2.4326, 78.8978) (2.4326, 78.6061) (2.744, 78.3243) (3.09, 78.2354) knots 0 0 0 1 2 2 2
  spline S27 degree 2 poles (3.09, 78.2354) (3.2581, 78.1909) (3.6832, 78.1019) (3.9156, 78.0475) knots 0 0 0 1 2 2 2
  spline S28 degree 2 poles (3.9156, 78.0475) (4.4198, 77.919) (4.9339, 77.3307) (4.9339, 76.8216) knots 0 0 0 1 2 2 2
  spline S29 degree 2 poles (4.9339, 76.8216) (4.9339, 76.525) (4.7015, 76.001) (4.4742, 75.8082) knots 0 0 0 1 2 2 2
  spline S30 degree 2 poles (4.4742, 75.8082) (4.2319, 75.6055) (3.614, 75.393) (3.1444, 75.393) knots 0 0 0 1 2 2 2
  line L28 (6.4366, 75.5017) -> (5.6655, 75.5017)
  line L29 (5.6655, 75.5017) -> (5.6655, 80.0792)
  line L30 (5.6655, 80.0792) -> (6.4366, 80.0792)
  line L31 (6.4366, 80.0792) -> (6.4366, 75.5017)
  line L32 (6.491, 80.8405) -> (5.616, 80.8405)
  line L33 (5.616, 80.8405) -> (5.616, 81.6413)
  line L34 (5.616, 81.6413) -> (6.491, 81.6413)
  line L35 (6.491, 81.6413) -> (6.491, 80.8405)
  line L36 (11.1624, 75.5017) -> (10.3912, 75.5017)
  line L37 (10.3912, 75.5017) -> (10.3912, 78.1118)
  spline S31 degree 2 poles (10.3912, 78.1118) (10.3912, 78.4282) (10.3319, 78.9719) (10.243, 79.135) knots 0 0 0 1 2 2 2
  spline S32 degree 2 poles (10.243, 79.135) (10.149, 79.3081) (9.8129, 79.4761) (9.5262, 79.4761) knots 0 0 0 1 2 2 2
  spline S33 degree 2 poles (9.5262, 79.4761) (9.2395, 79.4761) (8.6314, 79.1696) (8.3398, 78.9225) knots 0 0 0 1 2 2 2
  line L38 (8.3398, 78.9225) -> (8.3398, 75.5017)
  line L39 (8.3398, 75.5017) -> (7.5686, 75.5017)
  line L40 (7.5686, 75.5017) -> (7.5686, 80.0792)
  line L41 (7.5686, 80.0792) -> (8.3398, 80.0792)
  line L42 (8.3398, 80.0792) -> (8.3398, 79.57)
  spline S34 degree 2 poles (8.3398, 79.57) (8.6858, 79.8815) (9.3532, 80.2077) (9.7289, 80.2077) knots 0 0 0 1 2 2 2
  spline S35 degree 2 poles (9.7289, 80.2077) (10.4011, 80.2077) (11.1624, 79.3179) (11.1624, 78.4726) knots 0 0 0 1 2 2 2
  line L43 (11.1624, 78.4726) -> (11.1624, 75.5017)
  spline S36 degree 2 poles (12.4081, 74.7701) (12.4872, 74.7355) (12.7887, 74.6268) (12.9815, 74.5823) knots 0 0 0 1 2 2 2
  spline S37 degree 2 poles (12.9815, 74.5823) (13.1941, 74.5279) (13.5549, 74.4636) (13.7675, 74.4636) knots 0 0 0 1 2 2 2
  spline S38 degree 2 poles (13.7675, 74.4636) (14.1234, 74.4636) (14.6177, 74.6515) (14.7562, 74.8196) knots 0 0 0 1 2 2 2
  spline S39 degree 2 poles (14.7562, 74.8196) (14.8896, 74.9876) (14.9934, 75.4276) (14.9934, 75.7093) knots 0 0 0 1 2 2 2
  line L44 (14.9934, 75.7093) -> (14.9934, 76.1098)
  spline S40 degree 2 poles (14.9934, 76.1098) (14.682, 75.8379) (14.0839, 75.5808) (13.634, 75.5808) knots 0 0 0 1 2 2 2
  spline S41 degree 2 poles (13.634, 75.5808) (12.853, 75.5808) (11.9286, 76.7425) (11.9286, 77.835) knots 0 0 0 1 2 2 2
  spline S42 degree 2 poles (11.9286, 77.835) (11.9286, 78.4034) (12.2499, 79.2833) (12.5169, 79.5948) knots 0 0 0 1 2 2 2
  spline S43 degree 2 poles (12.5169, 79.5948) (12.7739, 79.8864) (13.4808, 80.2077) (13.8565, 80.2077) knots 0 0 0 1 2 2 2
  spline S44 degree 2 poles (13.8565, 80.2077) (14.2124, 80.2077) (14.7314, 80.0397) (14.9934, 79.8864) knots 0 0 0 1 2 2 2
  line L45 (14.9934, 79.8864) -> (15.0379, 80.0792)
  line L46 (15.0379, 80.0792) -> (15.7646, 80.0792)
  line L47 (15.7646, 80.0792) -> (15.7646, 76.0257)
  spline S45 degree 2 poles (15.7646, 76.0257) (15.7646, 74.8591) (14.7512, 73.7716) (13.7082, 73.7716) knots 0 0 0 1 2 2 2
  spline S46 degree 2 poles (13.7082, 73.7716) (13.372, 73.7716) (12.6701, 73.8803) (12.3686, 73.9693) knots 0 0 0 1 2 2 2
  line L48 (12.3686, 73.9693) -> (12.3686, 74.7701)
  line L49 (12.3686, 74.7701) -> (12.4081, 74.7701)
  line L50 (14.9934, 76.7425) -> (14.9934, 79.2586)
  spline S47 degree 2 poles (14.9934, 79.2586) (14.7067, 79.397) (14.2223, 79.5157) (13.9801, 79.5157) knots 0 0 0 1 2 2 2
  spline S48 degree 2 poles (13.9801, 79.5157) (13.3968, 79.5157) (12.7245, 78.6555) (12.7245, 77.8498) knots 0 0 0 1 2 2 2
  spline S49 degree 2 poles (12.7245, 77.8498) (12.7245, 77.0885) (13.2336, 76.2927) (13.8071, 76.2927) knots 0 0 0 1 2 2 2
  spline S50 degree 2 poles (13.8071, 76.2927) (14.1086, 76.2927) (14.7413, 76.5299) (14.9934, 76.7425) knots 0 0 0 1 2 2 2
  spline S51 degree 2 poles (-10.4348, 65.9427) (-10.5287, 65.8735) (-10.8451, 65.6263) (-10.9934, 65.5522) knots 0 0 0 1 2 2 2
  spline S52 degree 2 poles (-10.9934, 65.5522) (-11.196, 65.4434) (-11.5767, 65.3297) (-11.9227, 65.3297) knots 0 0 0 1 2 2 2
  spline S53 degree 2 poles (-11.9227, 65.3297) (-12.2045, 65.3297) (-12.7136, 65.5423) (-12.9064, 65.7351) knots 0 0 0 1 2 2 2
  spline S54 degree 2 poles (-12.9064, 65.7351) (-13.0893, 65.9229) (-13.3117, 66.4766) (-13.3117, 66.783) knots 0 0 0 1 2 2 2
  spline S55 degree 2 poles (-13.3117, 66.783) (-13.3117, 67.2576) (-12.9113, 67.9299) (-12.4763, 68.1227) knots 0 0 0 1 2 2 2
  spline S56 degree 2 poles (-12.4763, 68.1227) (-12.0908, 68.3006) (-11.0428, 68.4341) (-10.4348, 68.4687) knots 0 0 0 1 2 2 2
  line L51 (-10.4348, 68.4687) -> (-10.4348, 68.617)
  spline S57 degree 2 poles (-10.4348, 68.617) (-10.4348, 68.8839) (-10.5979, 69.2151) (-10.7462, 69.3091) knots 0 0 0 1 2 2 2
  spline S58 degree 2 poles (-10.7462, 69.3091) (-10.8945, 69.403) (-11.3196, 69.4623) (-11.547, 69.4623) knots 0 0 0 1 2 2 2
  spline S59 degree 2 poles (-11.547, 69.4623) (-11.8139, 69.4623) (-12.5357, 69.3041) (-12.8965, 69.1509) knots 0 0 0 1 2 2 2
  line L52 (-12.8965, 69.1509) -> (-12.941, 69.1509)
  line L53 (-12.941, 69.1509) -> (-12.941, 69.9368)
  spline S60 degree 2 poles (-12.941, 69.9368) (-12.7284, 69.9962) (-11.9326, 70.1445) (-11.5421, 70.1445) knots 0 0 0 1 2 2 2
  spline S61 degree 2 poles (-11.5421, 70.1445) (-11.0675, 70.1445) (-10.4199, 69.9962) (-10.1629, 69.8034) knots 0 0 0 1 2 2 2
  spline S62 degree 2 poles (-10.1629, 69.8034) (-9.9108, 69.6155) (-9.6636, 69.0174) (-9.6636, 68.5873) knots 0 0 0 1 2 2 2
  line L54 (-9.6636, 68.5873) -> (-9.6636, 65.4582)
  line L55 (-9.6636, 65.4582) -> (-10.4348, 65.4582)
  line L56 (-10.4348, 65.4582) -> (-10.4348, 65.9427)
  line L57 (-10.4348, 66.5853) -> (-10.4348, 67.8557)
  spline S63 degree 2 poles (-10.4348, 67.8557) (-10.7116, 67.831) (-11.547, 67.747) (-11.809, 67.6679) knots 0 0 0 1 2 2 2
  spline S64 degree 2 poles (-11.809, 67.6679) (-12.1155, 67.574) (-12.5159, 67.1834) (-12.5159, 66.8374) knots 0 0 0 1 2 2 2
  spline S65 degree 2 poles (-12.5159, 66.8374) (-12.5159, 66.442) (-12.071, 66.0415) (-11.6459, 66.0415) knots 0 0 0 1 2 2 2
  spline S66 degree 2 poles (-11.6459, 66.0415) (-11.285, 66.0415) (-10.6918, 66.353) (-10.4348, 66.5853) knots 0 0 0 1 2 2 2
  line L58 (-4.9873, 65.4582) -> (-5.7584, 65.4582)
  line L59 (-5.7584, 65.4582) -> (-5.7584, 68.0683)
  spline S67 degree 2 poles (-5.7584, 68.0683) (-5.7584, 68.3847) (-5.8177, 68.9284) (-5.9067, 69.0915) knots 0 0 0 1 2 2 2
  spline S68 degree 2 poles (-5.9067, 69.0915) (-6.0006, 69.2646) (-6.3368, 69.4326) (-6.6235, 69.4326) knots 0 0 0 1 2 2 2
  spline S69 degree 2 poles (-6.6235, 69.4326) (-6.9102, 69.4326) (-7.5182, 69.1262) (-7.8099, 68.879) knots 0 0 0 1 2 2 2
  line L60 (-7.8099, 68.879) -> (-7.8099, 65.4582)
  line L61 (-7.8099, 65.4582) -> (-8.581, 65.4582)
  line L62 (-8.581, 65.4582) -> (-8.581, 70.0357)
  line L63 (-8.581, 70.0357) -> (-7.8099, 70.0357)
  line L64 (-7.8099, 70.0357) -> (-7.8099, 69.5266)
  spline S70 degree 2 poles (-7.8099, 69.5266) (-7.4639, 69.838) (-6.7965, 70.1642) (-6.4208, 70.1642) knots 0 0 0 1 2 2 2
  spline S71 degree 2 poles (-6.4208, 70.1642) (-5.7485, 70.1642) (-4.9873, 69.2744) (-4.9873, 68.4291) knots 0 0 0 1 2 2 2
  line L65 (-4.9873, 68.4291) -> (-4.9873, 65.4582)
  line L66 (-0.3851, 65.4582) -> (-1.1562, 65.4582)
  line L67 (-1.1562, 65.4582) -> (-1.1562, 65.9229)
  spline S72 degree 2 poles (-1.1562, 65.9229) (-1.3342, 65.7746) (-1.5962, 65.5769) (-1.7741, 65.4928) knots 0 0 0 1 2 2 2
  spline S73 degree 2 poles (-1.7741, 65.4928) (-1.9373, 65.4138) (-2.2882, 65.3297) (-2.5206, 65.3297) knots 0 0 0 1 2 2 2
  spline S74 degree 2 poles (-2.5206, 65.3297) (-2.8963, 65.3297) (-3.529, 65.6411) (-3.7515, 65.9427) knots 0 0 0 1 2 2 2
  spline S75 degree 2 poles (-3.7515, 65.9427) (-3.9739, 66.2442) (-4.2211, 67.134) (-4.2211, 67.7124) knots 0 0 0 1 2 2 2
  spline S76 degree 2 poles (-4.2211, 67.7124) (-4.2211, 68.3155) (-3.9096, 69.1954) (-3.6378, 69.5266) knots 0 0 0 1 2 2 2
  spline S77 degree 2 poles (-3.6378, 69.5266) (-3.3857, 69.8232) (-2.6788, 70.1642) (-2.2882, 70.1642) knots 0 0 0 1 2 2 2
  spline S78 degree 2 poles (-2.2882, 70.1642) (-1.9472, 70.1642) (-1.438, 70.011) (-1.1562, 69.8528) knots 0 0 0 1 2 2 2
  line L68 (-1.1562, 69.8528) -> (-1.1562, 71.8301)
  line L69 (-1.1562, 71.8301) -> (-0.3851, 71.8301)
  line L70 (-0.3851, 71.8301) -> (-0.3851, 65.4582)
  line L71 (-1.1562, 66.5705) -> (-1.1562, 69.2151)
  spline S79 degree 2 poles (-1.1562, 69.2151) (-1.4429, 69.3535) (-1.8977, 69.4574) (-2.1597, 69.4574) knots 0 0 0 1 2 2 2
  spline S80 degree 2 poles (-2.1597, 69.4574) (-2.7529, 69.4574) (-3.4252, 68.5676) (-3.4252, 67.7272) knots 0 0 0 1 2 2 2
  spline S81 degree 2 poles (-3.4252, 67.7272) (-3.4252, 66.9165) (-2.9111, 66.0613) (-2.3426, 66.0613) knots 0 0 0 1 2 2 2
  spline S82 degree 2 poles (-2.3426, 66.0613) (-2.0411, 66.0613) (-1.4281, 66.3381) (-1.1562, 66.5705) knots 0 0 0 1 2 2 2
  spline S83 degree 2 poles (7.5489, 67.3317) (7.5489, 66.877) (7.2028, 66.18) (6.9161, 65.9526) knots 0 0 0 1 2 2 2
  spline S84 degree 2 poles (6.9161, 65.9526) (6.5701, 65.6856) (5.7841, 65.4582) (5.1613, 65.4582) knots 0 0 0 1 2 2 2
  line L72 (5.1613, 65.4582) -> (3.4113, 65.4582)
  line L73 (3.4113, 65.4582) -> (3.4113, 71.5582)
  line L74 (3.4113, 71.5582) -> (5.0278, 71.5582)
  spline S85 degree 2 poles (5.0278, 71.5582) (5.6803, 71.5582) (6.3328, 71.4742) (6.6294, 71.3111) knots 0 0 0 1 2 2 2
  spline S86 degree 2 poles (6.6294, 71.3111) (6.9606, 71.1381) (7.2622, 70.5696) (7.2622, 70.184) knots 0 0 0 1 2 2 2
  spline S87 degree 2 poles (7.2622, 70.184) (7.2622, 69.7539) (6.8074, 69.0718) (6.407, 68.879) knots 0 0 0 1 2 2 2
  line L75 (6.407, 68.879) -> (6.407, 68.8493)
  spline S88 degree 2 poles (6.407, 68.8493) (6.9507, 68.701) (7.5489, 67.915) (7.5489, 67.3317) knots 0 0 0 1 2 2 2
  spline S89 degree 2 poles (6.7036, 67.2971) (6.7036, 67.6432) (6.5058, 68.0881) (6.2092, 68.2462) knots 0 0 0 1 2 2 2
  spline S90 degree 2 poles (6.2092, 68.2462) (6.0165, 68.3451) (5.5617, 68.4044) (5.1415, 68.4044) knots 0 0 0 1 2 2 2
  line L76 (5.1415, 68.4044) -> (4.222, 68.4044)
  line L77 (4.222, 68.4044) -> (4.222, 66.1503)
  line L78 (4.222, 66.1503) -> (4.8795, 66.1503)
  spline S91 degree 2 poles (4.8795, 66.1503) (5.4134, 66.1503) (6.0263, 66.2492) (6.2636, 66.4074) knots 0 0 0 1 2 2 2
  spline S92 degree 2 poles (6.2636, 66.4074) (6.491, 66.5705) (6.7036, 66.9758) (6.7036, 67.2971) knots 0 0 0 1 2 2 2
  spline S93 degree 2 poles (6.4169, 70.0703) (6.4169, 70.2878) (6.2686, 70.6141) (6.1054, 70.708) knots 0 0 0 1 2 2 2
  spline S94 degree 2 poles (6.1054, 70.708) (5.9077, 70.8168) (5.4282, 70.8662) (4.9981, 70.8662) knots 0 0 0 1 2 2 2
  line L79 (4.9981, 70.8662) -> (4.222, 70.8662)
  line L80 (4.222, 70.8662) -> (4.222, 69.0817)
  line L81 (4.222, 69.0817) -> (5.1415, 69.0817)
  spline S95 degree 2 poles (5.1415, 69.0817) (5.5221, 69.0817) (5.883, 69.1608) (6.0758, 69.2843) knots 0 0 0 1 2 2 2
  spline S96 degree 2 poles (6.0758, 69.2843) (6.2636, 69.403) (6.4169, 69.7836) (6.4169, 70.0703) knots 0 0 0 1 2 2 2
  line L82 (10.7224, 69.2102) -> (10.6829, 69.2102)
  spline S97 degree 2 poles (10.6829, 69.2102) (10.5939, 69.2349) (10.4011, 69.2448) (10.2677, 69.2448) knots 0 0 0 1 2 2 2
  spline S98 degree 2 poles (10.2677, 69.2448) (9.9562, 69.2448) (9.3433, 68.9729) (9.0665, 68.706) knots 0 0 0 1 2 2 2
  line L83 (9.0665, 68.706) -> (9.0665, 65.4582)
  line L84 (9.0665, 65.4582) -> (8.2953, 65.4582)
  line L85 (8.2953, 65.4582) -> (8.2953, 70.0357)
  line L86 (8.2953, 70.0357) -> (9.0665, 70.0357)
  line L87 (9.0665, 70.0357) -> (9.0665, 69.3535)
  spline S99 degree 2 poles (9.0665, 69.3535) (9.4866, 69.7292) (10.1144, 70.0357) (10.411, 70.0357) knots 0 0 0 1 2 2 2
  spline S100 degree 2 poles (10.411, 70.0357) (10.5297, 70.0357) (10.6483, 70.0258) (10.7224, 70.011) knots 0 0 0 1 2 2 2
  line L88 (10.7224, 70.011) -> (10.7224, 69.2102)
  spline S101 degree 2 poles (13.8713, 65.9427) (13.7774, 65.8735) (13.461, 65.6263) (13.3127, 65.5522) knots 0 0 0 1 2 2 2
  spline S102 degree 2 poles (13.3127, 65.5522) (13.1101, 65.4434) (12.7294, 65.3297) (12.3834, 65.3297) knots 0 0 0 1 2 2 2
  spline S103 degree 2 poles (12.3834, 65.3297) (12.1016, 65.3297) (11.5925, 65.5423) (11.3997, 65.7351) knots 0 0 0 1 2 2 2
  spline S104 degree 2 poles (11.3997, 65.7351) (11.2168, 65.9229) (10.9943, 66.4766) (10.9943, 66.783) knots 0 0 0 1 2 2 2
  spline S105 degree 2 poles (10.9943, 66.783) (10.9943, 67.2576) (11.3947, 67.9299) (11.8297, 68.1227) knots 0 0 0 1 2 2 2
  spline S106 degree 2 poles (11.8297, 68.1227) (12.2153, 68.3006) (13.2633, 68.4341) (13.8713, 68.4687) knots 0 0 0 1 2 2 2
  line L89 (13.8713, 68.4687) -> (13.8713, 68.617)
  spline S107 degree 2 poles (13.8713, 68.617) (13.8713, 68.8839) (13.7082, 69.2151) (13.5599, 69.3091) knots 0 0 0 1 2 2 2
  spline S108 degree 2 poles (13.5599, 69.3091) (13.4116, 69.403) (12.9865, 69.4623) (12.7591, 69.4623) knots 0 0 0 1 2 2 2
  spline S109 degree 2 poles (12.7591, 69.4623) (12.4921, 69.4623) (11.7704, 69.3041) (11.4096, 69.1509) knots 0 0 0 1 2 2 2
  line L90 (11.4096, 69.1509) -> (11.3651, 69.1509)
  line L91 (11.3651, 69.1509) -> (11.3651, 69.9368)
  spline S110 degree 2 poles (11.3651, 69.9368) (11.5776, 69.9962) (12.3735, 70.1445) (12.764, 70.1445) knots 0 0 0 1 2 2 2
  spline S111 degree 2 poles (12.764, 70.1445) (13.2386, 70.1445) (13.8861, 69.9962) (14.1432, 69.8034) knots 0 0 0 1 2 2 2
  spline S112 degree 2 poles (14.1432, 69.8034) (14.3953, 69.6155) (14.6425, 69.0174) (14.6425, 68.5873) knots 0 0 0 1 2 2 2
  line L92 (14.6425, 68.5873) -> (14.6425, 65.4582)
  line L93 (14.6425, 65.4582) -> (13.8713, 65.4582)
  line L94 (13.8713, 65.4582) -> (13.8713, 65.9427)
  line L95 (13.8713, 66.5853) -> (13.8713, 67.8557)
  spline S113 degree 2 poles (13.8713, 67.8557) (13.5945, 67.831) (12.7591, 67.747) (12.4971, 67.6679) knots 0 0 0 1 2 2 2
  spline S114 degree 2 poles (12.4971, 67.6679) (12.1906, 67.574) (11.7902, 67.1834) (11.7902, 66.8374) knots 0 0 0 1 2 2 2
  spline S115 degree 2 poles (11.7902, 66.8374) (11.7902, 66.442) (12.2351, 66.0415) (12.6602, 66.0415) knots 0 0 0 1 2 2 2
  spline S116 degree 2 poles (12.6602, 66.0415) (13.0211, 66.0415) (13.6143, 66.353) (13.8713, 66.5853) knots 0 0 0 1 2 2 2
  spline S117 degree 2 poles (17.5442, 65.3544) (17.0696, 65.3544) (16.2836, 65.6461) (16.0019, 65.9427) knots 0 0 0 1 2 2 2
  spline S118 degree 2 poles (16.0019, 65.9427) (15.7201, 66.2343) (15.4087, 67.134) (15.4087, 67.7371) knots 0 0 0 1 2 2 2
  spline S119 degree 2 poles (15.4087, 67.7371) (15.4087, 68.3402) (15.73, 69.2201) (16.0019, 69.5167) knots 0 0 0 1 2 2 2
  spline S120 degree 2 poles (16.0019, 69.5167) (16.2737, 69.8182) (17.0795, 70.1395) (17.5442, 70.1395) knots 0 0 0 1 2 2 2
  spline S121 degree 2 poles (17.5442, 70.1395) (17.9199, 70.1395) (18.6218, 69.927) (18.8937, 69.7885) knots 0 0 0 1 2 2 2
  line L96 (18.8937, 69.7885) -> (18.8937, 68.9235)
  line L97 (18.8937, 68.9235) -> (18.8492, 68.9235)
  spline S122 degree 2 poles (18.8492, 68.9235) (18.7652, 68.9927) (18.5081, 69.1706) (18.3252, 69.2646) knots 0 0 0 1 2 2 2
  spline S123 degree 2 poles (18.3252, 69.2646) (18.1621, 69.3437) (17.7271, 69.4672) (17.5293, 69.4672) knots 0 0 0 1 2 2 2
  spline S124 degree 2 poles (17.5293, 69.4672) (16.9312, 69.4672) (16.2045, 68.5626) (16.2045, 67.7371) knots 0 0 0 1 2 2 2
  spline S125 degree 2 poles (16.2045, 67.7371) (16.2045, 66.9313) (16.9065, 66.0267) (17.5293, 66.0267) knots 0 0 0 1 2 2 2
  spline S126 degree 2 poles (17.5293, 66.0267) (17.905, 66.0267) (18.5872, 66.3381) (18.8492, 66.5804) knots 0 0 0 1 2 2 2
  line L98 (18.8492, 66.5804) -> (18.8937, 66.5804)
  line L99 (18.8937, 66.5804) -> (18.8937, 65.7153)
  spline S127 degree 2 poles (18.8937, 65.7153) (18.78, 65.6609) (18.434, 65.5077) (18.2955, 65.4731) knots 0 0 0 1 2 2 2
  spline S128 degree 2 poles (18.2955, 65.4731) (18.0978, 65.4138) (17.7864, 65.3544) (17.5442, 65.3544) knots 0 0 0 1 2 2 2
  line L100 (23.3871, 65.4582) -> (22.3737, 65.4582)
  line L101 (22.3737, 65.4582) -> (20.6733, 67.6679)
  line L102 (20.6733, 67.6679) -> (20.3668, 67.3713)
  line L103 (20.3668, 67.3713) -> (20.3668, 65.4582)
  line L104 (20.3668, 65.4582) -> (19.5956, 65.4582)
  line L105 (19.5956, 65.4582) -> (19.5956, 71.8301)
  line L106 (19.5956, 71.8301) -> (20.3668, 71.8301)
  line L107 (20.3668, 71.8301) -> (20.3668, 68.1029)
  line L108 (20.3668, 68.1029) -> (22.176, 70.0357)
  line L109 (22.176, 70.0357) -> (23.135, 70.0357)
  line L110 (23.135, 70.0357) -> (21.2566, 68.1227)
  line L111 (21.2566, 68.1227) -> (23.3871, 65.4582)
  spline S129 degree 2 poles (25.7599, 65.3544) (24.6625, 65.3544) (23.4563, 66.5853) (23.4563, 67.7223) knots 0 0 0 1 2 2 2
  spline S130 degree 2 poles (23.4563, 67.7223) (23.4563, 68.8394) (24.6279, 70.1642) (25.572, 70.1642) knots 0 0 0 1 2 2 2
  spline S131 degree 2 poles (25.572, 70.1642) (25.9972, 70.1642) (26.6546, 69.9171) (26.8968, 69.6551) knots 0 0 0 1 2 2 2
  spline S132 degree 2 poles (26.8968, 69.6551) (27.144, 69.3931) (27.406, 68.6368) (27.406, 68.0881) knots 0 0 0 1 2 2 2
  line L112 (27.406, 68.0881) -> (27.406, 67.6679)
  line L113 (27.406, 67.6679) -> (24.2374, 67.6679)
  spline S133 degree 2 poles (24.2374, 67.6679) (24.2374, 66.872) (25.0382, 66.0267) (25.75, 66.0267) knots 0 0 0 1 2 2 2
  spline S134 degree 2 poles (25.75, 66.0267) (26.0021, 66.0267) (26.4915, 66.1404) (26.6892, 66.2294) knots 0 0 0 1 2 2 2
  spline S135 degree 2 poles (26.6892, 66.2294) (26.8968, 66.3283) (27.1836, 66.5013) (27.2775, 66.5804) knots 0 0 0 1 2 2 2
  line L114 (27.2775, 66.5804) -> (27.322, 66.5804)
  line L115 (27.322, 66.5804) -> (27.322, 65.74)
  spline S136 degree 2 poles (27.322, 65.74) (27.1885, 65.6856) (26.7831, 65.5274) (26.625, 65.483) knots 0 0 0 1 2 2 2
  spline S137 degree 2 poles (26.625, 65.483) (26.4025, 65.4187) (26.0367, 65.3544) (25.7599, 65.3544) knots 0 0 0 1 2 2 2
  spline S138 degree 2 poles (26.6546, 68.2561) (26.6447, 68.5676) (26.5162, 69.0223) (26.3926, 69.1756) knots 0 0 0 1 2 2 2
  spline S139 degree 2 poles (26.3926, 69.1756) (26.2592, 69.3486) (25.839, 69.5315) (25.5276, 69.5315) knots 0 0 0 1 2 2 2
  spline S140 degree 2 poles (25.5276, 69.5315) (25.2211, 69.5315) (24.791, 69.3486) (24.613, 69.1706) knots 0 0 0 1 2 2 2
  spline S141 degree 2 poles (24.613, 69.1706) (24.44, 68.9877) (24.2621, 68.5478) (24.2374, 68.2561) knots 0 0 0 1 2 2 2
  line L116 (24.2374, 68.2561) -> (26.6546, 68.2561)
  spline S142 degree 2 poles (29.5712, 65.3693) (28.9434, 65.3693) (28.2365, 66.086) (28.2365, 66.8621) knots 0 0 0 1 2 2 2
  line L117 (28.2365, 66.8621) -> (28.2365, 69.398)
  line L118 (28.2365, 69.398) -> (27.7174, 69.398)
  line L119 (27.7174, 69.398) -> (27.7174, 70.0357)
  line L120 (27.7174, 70.0357) -> (28.2365, 70.0357)
  line L121 (28.2365, 70.0357) -> (28.2365, 71.3506)
  line L122 (28.2365, 71.3506) -> (29.0076, 71.3506)
  line L123 (29.0076, 71.3506) -> (29.0076, 70.0357)
  line L124 (29.0076, 70.0357) -> (30.4263, 70.0357)
  line L125 (30.4263, 70.0357) -> (30.4263, 69.398)
  line L126 (30.4263, 69.398) -> (29.0076, 69.398)
  line L127 (29.0076, 69.398) -> (29.0076, 67.218)
  spline S143 degree 2 poles (29.0076, 67.218) (29.0076, 66.872) (29.0323, 66.4914) (29.1164, 66.3283) knots 0 0 0 1 2 2 2
  spline S144 degree 2 poles (29.1164, 66.3283) (29.1856, 66.1849) (29.497, 66.0415) (29.7639, 66.0415) knots 0 0 0 1 2 2 2
  spline S145 degree 2 poles (29.7639, 66.0415) (29.9518, 66.0415) (30.3028, 66.1552) (30.3818, 66.1898) knots 0 0 0 1 2 2 2
  line L128 (30.3818, 66.1898) -> (30.4263, 66.1898)
  line L129 (30.4263, 66.1898) -> (30.4263, 65.4978)
  spline S146 degree 2 poles (30.4263, 65.4978) (30.2088, 65.4385) (29.7639, 65.3693) (29.5712, 65.3693) knots 0 0 0 1 2 2 2
  point P0 (-122.1423, 0)
  constraints: 2 other
extrude "Extrusion40" cut sketch "Sketch39" against normal blind 0.5 bodies 1
ref_plane "Work Plane11" through (122.1423, 0, 0) normal (0, 0, 1) x (1, 0, 0)
equation "\"d12\" = d11"
equation "\"d13\" = d11"
equation "\"d14\" = d11"
equation "\"d15\" = d7"
equation "\"d19\" = d14"
equation "\"d20\" = d19"
equation "\"d21\" = d19"
equation "\"d22\" = d19"
equation "\"d26\" = d25"
equation "\"d27\" = d25"
equation "\"d28\" = d25"
equation "\"d31\" = d30"
equation "\"d33\" = d24"
equation "\"d34\" = d23"
equation "\"d35\" = d25"
equation "\"d36\" = d35"
equation "\"d37\" = d35"